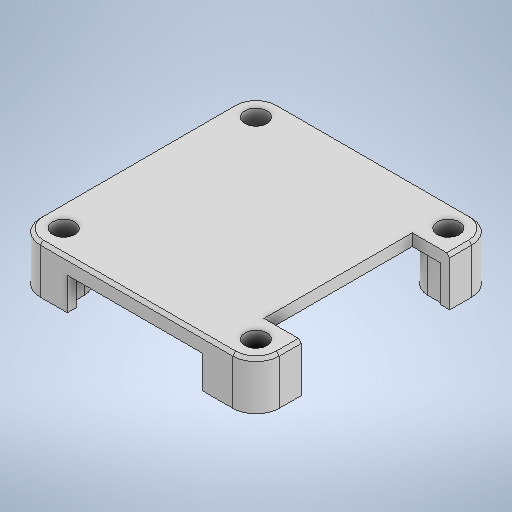
# Autodesk Inventor part: oDrive_micro_cover
Saved by Autodesk Inventor 2025.2 (Build 292293000, 293)
## iProperties
Created: 2025-05-11
Part Number: oDrive_micro_cover
Material: Generic
Document SubType Name: Modeling
Designer: Bruno
Density: 1 g/cm^3
Appearance: Default
Author: Bruno
## iProperties of the stored document oDrive_micro_cover_3DPrint.ipt
Created: 2025-05-11
Part Number: oDrive_micro_cover_3DPrint
Material: Generic
Document SubType Name: Modeling
Designer: Bruno
Density: 1 g/cm^3
Appearance: Default
Author: Bruno
Autodesk Inventor part; units mm, degrees
ref_plane "YZ Plane" through (0, 0, 0) normal (1, 0, 0) x (0, 1, 0)
ref_plane "XZ Plane" through (0, 0, 0) normal (0, 1, 0) x (-1, 0, 0)
ref_plane "XY Plane" through (0, 0, 0) normal (0, 0, 1) x (1, 0, 0)
sketch "Sketch1" plane through (0, 0, 0) normal (0, 1, 0) x (-1, 0, 0)
  line L0 (16.15, 16.15) -> (-16.15, 16.15)
  line L1 (-16.15, 16.15) -> (-16.15, -16.15)
  line L2 (-16.15, -16.15) -> (16.15, -16.15)
  line L3 (16.15, -16.15) -> (16.15, 16.15)
  line L4 (16.15, 16.15) -> (-16.15, -16.15) construction
  line L5 (-16.15, 16.15) -> (16.15, -16.15) construction
  arc A0 (16.15, 13) -> (13, 16.15) centre (13, 13) ccw
  arc A1 (-13, 16.15) -> (-16.15, 13) centre (-13, 13) ccw
  arc A2 (-16.15, -13) -> (-13, -16.15) centre (-13, -13) ccw
  arc A3 (13, -16.15) -> (16.15, -13) centre (13, -13) ccw
  point P0 (0, 0)
  point P1 (13, -16.15)
  point P2 (16.15, -13)
  point P3 (-13, 16.15)
  point P4 (-16.15, 13)
  point P5 (-16.15, -13)
  point P6 (-13, -16.15)
  dimension "d0" = 32.3
  dimension "d1" = 3.15
  dimension "d4" = 360
  constraints: 12 end point, 8 point on circle, 4 centre point, 2 midpoint, 2 parallel, 2 perpendicular, 2 point on line, 2 tangent, 1 horizontal, 17 other
  measures "d0" distance between parallel lines of L0 L2
  measures "d1" radius of A0
extrude "Extrusion1" add sketch "Sketch1" along normal blind 7 contours A0 L3 A3 L2 A2 L1 A1 L0
sketch "Sketch2" plane through (0, 7, 0) normal (0, 1, 0) x (1, 0, 0)
  line L0 (-16.15, 13) -> (-16.15, -13) projected
  arc A0 (-16.15, -13) -> (-13, -16.15) centre (-13, -13) ccw projected
  line L1 (-13, -16.15) -> (13, -16.15) projected
  arc A1 (13, -16.15) -> (16.15, -13) centre (13, -13) ccw projected
  line L2 (16.15, -13) -> (16.15, 13) projected
  arc A2 (16.15, 13) -> (13, 16.15) centre (13, 13) ccw projected
  line L3 (13, 16.15) -> (-13, 16.15) projected
  arc A3 (-13, 16.15) -> (-16.15, 13) centre (-13, 13) ccw projected
  line L4 (16.15, -10.025) -> (11.1, -10.025)
  line L5 (11.1, -10.025) -> (11.1, 10.025)
  line L6 (11.1, 10.025) -> (16.15, 10.025)
  line L7 (16.15, 0) -> (11.5552, 0) construction
  point P0 (0, 0)
  point P1 (13.625, -10.025)
  point P2 (11.1, 0)
  dimension "d8" = 5.05
  dimension "d10" = 20.05
  constraints: 8 end point, 3 midpoint, 2 horizontal, 2 perpendicular, 2 point on line, 1 horizontal alignment
  measures "d8" distance between parallel lines of L2 L5
  measures "d10" distance from line of point (13.625, -10.025) L6
extrude "Extrusion2" cut sketch "Sketch2" against normal through all contours L2 L4 L5 L6
sketch "Sketch4" plane through (0, 0, 0) normal (0, -1, 0) x (1, 0, 0)
  line L0 (16.15, -10.025) -> (16.15, -13) projected
  arc A0 (13, -16.15) -> (16.15, -13) centre (13, -13) ccw projected
  line L1 (13, -16.15) -> (-13, -16.15) projected
  line L2 (16.15, 13) -> (16.15, 10.025) projected
  arc A1 (16.15, 13) -> (13, 16.15) centre (13, 13) ccw projected
  line L3 (-13, 16.15) -> (13, 16.15) projected
  arc A2 (-13, 16.15) -> (-16.15, 13) centre (-13, 13) ccw projected
  line L4 (-16.15, -13) -> (-16.15, 13) projected
  arc A3 (-16.15, -13) -> (-13, -16.15) centre (-13, -13) ccw projected
  line L5 (16.15, 13) -> (16.15, 10.025) projected
  arc A4 (14.95, 13) -> (13, 14.95) centre (13, 13) ccw
  line L6 (13, 14.95) -> (-13, 14.95)
  arc A5 (-13, 14.95) -> (-14.95, 13) centre (-13, 13) ccw
  line L7 (-14.95, 13) -> (-14.95, -13)
  arc A6 (-14.95, -13) -> (-13, -14.95) centre (-13, -13) ccw
  line L8 (-13, -14.95) -> (13, -14.95)
  arc A7 (13, -14.95) -> (14.95, -13) centre (13, -13) ccw
  line L9 (14.95, -13) -> (14.95, -10.025)
  line L10 (14.95, 13) -> (14.95, -10.025)
  point P0 (0, 0)
  dimension "d13" = 1.2
  constraints: 10 end point, 8 point on circle, 4 centre point, 1 collinear, 7 other
  measures "d13" distance between parallel lines of L1 L8
extrude "Extrusion3" cut sketch "Sketch4" against normal blind 6
sketch "Sketch5" plane through (0, 0, 0) normal (0, -1, 0) x (1, 0, 0)
  line L0 (14.95, 13) -> (14.95, 10.025) projected
  line L1 (14.95, 10.025) -> (16.15, 10.025) projected
  line L2 (16.15, 13) -> (16.15, 10.025) projected
  arc A0 (16.15, 13) -> (13, 16.15) centre (13, 13) ccw projected
  line L3 (-13, 16.15) -> (13, 16.15) projected
  arc A1 (-13, 16.15) -> (-16.15, 13) centre (-13, 13) ccw projected
  line L4 (-16.15, -13) -> (-16.15, 13) projected
  arc A2 (-16.15, -13) -> (-13, -16.15) centre (-13, -13) ccw projected
  line L5 (13, -16.15) -> (-13, -16.15) projected
  arc A3 (13, -16.15) -> (16.15, -13) centre (13, -13) ccw projected
  line L6 (16.15, -10.025) -> (16.15, -13) projected
  line L7 (16.15, -10.025) -> (14.95, -10.025) projected
  line L8 (14.95, -10.025) -> (14.95, -13) projected
  arc A4 (13, -14.95) -> (14.95, -13) centre (13, -13) ccw projected
  line L9 (13, -14.95) -> (-13, -14.95) projected
  arc A5 (-14.95, -13) -> (-13, -14.95) centre (-13, -13) ccw projected
  line L10 (-14.95, -13) -> (-14.95, 13) projected
  arc A6 (-13, 14.95) -> (-14.95, 13) centre (-13, 13) ccw projected
  line L11 (-13, 14.95) -> (13, 14.95) projected
  arc A7 (14.95, 13) -> (13, 14.95) centre (13, 13) ccw projected
  line L12 (-9.65, -16.15) -> (-9.65, -14.95)
  line L13 (9.55, -16.15) -> (9.55, -14.95)
  line L14 (-9.35, 14.95) -> (-9.35, 16.15)
  line L15 (8.95, 14.95) -> (8.95, 16.15)
  line L16 (-14.95, -9.175) -> (-16.15, -9.175)
  line L17 (-14.95, 0) -> (-14.0185, 0) construction
  line L18 (-14.95, 9.175) -> (-16.15, 9.175)
  point P0 (0, 0)
  dimension "d16" = 6.5
  dimension "d17" = 19.2
  dimension "d18" = 6.8
  dimension "d19" = 18.3
  dimension "d20" = 18.35
  constraints: 14 end point, 10 point on line, 5 perpendicular, 2 symmetric about line, 1 horizontal, 1 midpoint
  measures "d16" distance between parallel lines of L4 L12
  measures "d17" distance between parallel lines of L12 L13
  measures "d18" distance between parallel lines of L4 L14
  measures "d19" distance between parallel lines of L14 L15
  measures "d20" distance between parallel lines of L18 L16
extrude "Extrusion4" cut sketch "Sketch5" against normal blind 4.4 contours L11 L14 L3 L15 | L10 L16 L4 L18 | L9 L13 L5 L12
sketch "Sketch6" plane through (0, 6, 0) normal (0, -1, 0) x (1, 0, 0)
  line L0 (8.95, 16.15) -> (8.95, 14.95) projected
  line L1 (-9.35, 14.95) -> (-9.35, 16.15) projected
  line L2 (-16.15, 9.175) -> (-14.95, 9.175) projected
  line L3 (-16.15, -13) -> (-16.15, 13) projected
  line L4 (13, -16.15) -> (-13, -16.15) projected
  line L5 (-16.15, 0) -> (-5.5986, 0) construction
  line L6 (0, -16.15) -> (0, -5.693) construction
  circle A0 centre (13, 13) radius 2.75
  circle A1 centre (13, -13) radius 2.75
  circle A2 centre (-13, 13) radius 2.75
  circle A3 centre (-13, -13) radius 2.75
  line L7 (11.1, -10.025) -> (16.15, -10.025) projected
  line L8 (16.15, -10.025) -> (16.15, -13) projected
  arc A4 (13, -16.15) -> (16.15, -13) centre (13, -13) ccw projected
  line L9 (13, -16.15) -> (-13, -16.15) projected
  arc A5 (-16.15, -13) -> (-13, -16.15) centre (-13, -13) ccw projected
  line L10 (-16.15, -13) -> (-16.15, 13) projected
  arc A6 (-13, 16.15) -> (-16.15, 13) centre (-13, 13) ccw projected
  line L11 (-13, 16.15) -> (13, 16.15) projected
  arc A7 (16.15, 13) -> (13, 16.15) centre (13, 13) ccw projected
  line L12 (16.15, 13) -> (16.15, 10.025) projected
  line L13 (16.15, 10.025) -> (11.1, 10.025) projected
  line L14 (11.1, 10.025) -> (11.1, -10.025) projected
  line L15 (-10.25, -16.15) -> (-10.25, -13)
  line L16 (-13, -10.25) -> (-16.15, -10.25)
  line L17 (13, -10.25) -> (16.15, -10.25)
  line L18 (10.25, -13) -> (10.25, -16.15)
  line L19 (13, 10.25) -> (16.15, 10.25)
  line L20 (10.25, 13) -> (10.25, 16.15)
  line L21 (-10.25, 13) -> (-10.25, 16.15)
  line L22 (-13, 10.25) -> (-16.15, 10.25)
  line L23 (14.95, 10.025) -> (11.1, 10.025) projected
  line L24 (14.95, 13) -> (14.95, 10.025) projected
  arc A8 (14.95, 13) -> (13, 14.95) centre (13, 13) ccw projected
  line L25 (-13, 14.95) -> (13, 14.95) projected
  arc A9 (-13, 14.95) -> (-14.95, 13) centre (-13, 13) ccw projected
  line L26 (-14.95, -13) -> (-14.95, 13) projected
  arc A10 (-14.95, -13) -> (-13, -14.95) centre (-13, -13) ccw projected
  line L27 (13, -14.95) -> (-13, -14.95) projected
  arc A11 (13, -14.95) -> (14.95, -13) centre (13, -13) ccw projected
  line L28 (14.95, -10.025) -> (14.95, -13) projected
  line L29 (11.1, -10.025) -> (14.95, -10.025) projected
  line L30 (11.1, 10.025) -> (11.1, -10.025) projected
  point P0 (0, 0)
  point P1 (14.95, -10.25)
  point P2 (10.25, -14.95)
  point P3 (-14.95, -10.25)
  point P4 (-10.25, -14.95)
  point P5 (-10.25, 14.95)
  point P6 (-14.95, 10.25)
  point P7 (10.25, 14.95)
  point P8 (14.95, 10.25)
  dimension "d48" = 5.5
  dimension "d49" = 26
  dimension "d50" = 26
  constraints: 20 end point, 10 point on line, 8 point on circle, 7 perpendicular, 7 tangent, 4 centre point, 3 symmetric about line, 2 midpoint, 1 horizontal, 1 vertical, 3 other
  measures "d48" diameter of A0
  measures "d49" distance of A1.centre A0.centre
  measures "d50" distance of A2.centre A0.centre
extrude "Extrusion5" add sketch "Sketch6" along normal up to surface (6 mm away) contours L25 A0 L20 | L21 A2 L25 | A0 L25 A8 L24 | A2 L26 A9 L25 | A0 L24 L19 | L22 L26 A2 | L16 A3 L26 | A3 L27 A10 L26 | L15 L27 A3 | L28 A1 L17 | A1 L28 A11 L27 | L18 A1 L27 picked at (13.0785, 12.9333) picked at (-13.0785, 12.9333) picked at (-12.9333, -13.0785) picked at (12.9333, -13.0785)
sketch "Sketch7" plane through (0, 0, 0) normal (0, -1, 0) x (1, 0, 0)
  circle A0 centre (13, 13) radius 1.5
  line L0 (-16.15, -13) -> (-16.15, 13) projected
  line L1 (13, -16.15) -> (-13, -16.15) projected
  line L2 (0, -16.15) -> (0, -7.7699) construction
  line L3 (-16.15, 0) -> (-9.6467, 0) construction
  circle A1 centre (13, -13) radius 1.5
  circle A2 centre (-13, 13) radius 1.5
  circle A3 centre (-13, -13) radius 1.5
  point P0 (0, 0)
  dimension "d31" = 3
  dimension "d41" = 26
  dimension "d42" = 26
  constraints: 4 centre point, 4 end point, 3 symmetric about line, 2 midpoint, 1 horizontal, 1 vertical, 3 other
  measures "d31" diameter of A0
  measures "d41" distance of A1.centre A0.centre
  measures "d42" distance of A3.centre A1.centre
extrude "Extrusion6" cut sketch "Sketch7" against normal through all
sketch "Sketch9" plane through (0, 6, 0) normal (0, -1, 0) x (1, 0, 0)
  line L0 (11.1, -10.025) -> (14.95, -10.025) projected
  line L1 (11.1, 10.025) -> (11.1, -10.025) projected
  line L2 (14.95, 10.025) -> (11.1, 10.025) projected
  line L3 (-10.25, 14.95) -> (10.25, 14.95) projected
  line L4 (-14.95, -10.25) -> (-14.95, 10.25) projected
  line L5 (10.25, -14.95) -> (-10.25, -14.95) projected
  line L6 (14.95, 10.25) -> (14.95, 10.025) projected
  line L7 (14.95, -10.025) -> (14.95, -10.25) projected
  line L8 (-10.25, -13) -> (-10.25, -14.95) projected
  line L9 (10.25, -14.95) -> (10.25, -13) projected
  arc A0 (13, -10.25) -> (10.25, -13) centre (13, -13) ccw projected
  line L10 (13, -10.25) -> (14.95, -10.25) projected
  line L11 (14.95, 10.25) -> (13, 10.25) projected
  arc A1 (10.25, 13) -> (13, 10.25) centre (13, 13) ccw projected
  line L12 (10.25, 13) -> (10.25, 14.95) projected
  line L13 (-10.25, 14.95) -> (-10.25, 13) projected
  arc A2 (-13, 10.25) -> (-10.25, 13) centre (-13, 13) ccw projected
  line L14 (-13, 10.25) -> (-14.95, 10.25) projected
  line L15 (-14.95, -10.25) -> (-13, -10.25) projected
  arc A3 (-10.25, -13) -> (-13, -10.25) centre (-13, -13) ccw projected
  point P0 (0, 0)
extrude "Extrusion8" add sketch "Sketch9" along normal blind 1.1
sketch "Sketch10" plane through (0, 7, 0) normal (0, 1, 0) x (1, 0, 0)
  circle A0 centre (-13, 13) radius 1.5 projected
  circle A1 centre (13, 13) radius 1.5 projected
  circle A2 centre (13, -13) radius 1.5 projected
  circle A3 centre (-13, -13) radius 1.5 projected
  line L0 (11.1, 10.025) -> (16.15, 10.025) projected
  line L1 (16.15, 10.025) -> (16.15, 13) projected
  arc A4 (16.15, 13) -> (13, 16.15) centre (13, 13) ccw projected
  line L2 (13, 16.15) -> (-13, 16.15) projected
  arc A5 (-13, 16.15) -> (-16.15, 13) centre (-13, 13) ccw projected
  line L3 (-16.15, 13) -> (-16.15, -13) projected
  arc A6 (-16.15, -13) -> (-13, -16.15) centre (-13, -13) ccw projected
  line L4 (-13, -16.15) -> (13, -16.15) projected
  arc A7 (13, -16.15) -> (16.15, -13) centre (13, -13) ccw projected
  line L5 (16.15, -13) -> (16.15, -10.025) projected
  line L6 (16.15, -10.025) -> (11.1, -10.025) projected
  line L7 (11.1, -10.025) -> (11.1, 10.025) projected
  point P0 (0, 0)
extrude "Extrusion9" cut sketch "Sketch10" against normal blind 0.5
sketch "Sketch11" plane through (0, 0, 0) normal (0, -1, 0) x (1, 0, 0)
  point P0 (0, 0)
chamfer "Chamfer2" distance 0.4 angle 45 9 edges at (0, 6.5, -16.15) (15.2274, 6.5, -15.2274) (16.15, 6.5, -11.5125) (-15.2274, 6.5, -15.2274) (-16.15, 6.5, 0) (-15.2274, 6.5, 15.2274) (0, 6.5, 16.15) (15.2274, 6.5, 15.2274) (16.15, 6.5, 11.5125)
body "Solid1"
